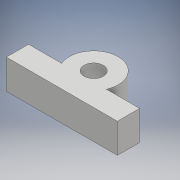
# Autodesk Inventor part: Mount for exis
Saved by Autodesk Inventor 2018 (Build 220112000, 112)
## iProperties
Created: 2019-04-02
Part Number: Mount for exis
Material: Типовые
Document SubType Name: Modeling
Designer: cosko
Density: 1 g/cm^3
Appearance: По умолчанию
Author: cosko
Autodesk Inventor part; units mm, degrees
ref_plane "YZ Plane" through (0, 0, 0) normal (1, 0, 0) x (0, 1, 0)
ref_plane "XZ Plane" through (0, 0, 0) normal (0, 1, 0) x (-1, 0, 0)
ref_plane "XY Plane" through (0, 0, 0) normal (0, 0, 1) x (1, 0, 0)
sketch "Эскиз1" plane through (0, 0, 0) normal (0, 0, 1) x (1, 0, 0)
  line L0 (0, 0) -> (0, 3) construction
  line L1 (0, 3) -> (2.6556, 3) construction
  line L2 (0, 3) -> (0, 5.6) construction
  circle A0 centre (0, 4.3) radius 1.3
  circle A1 centre (0, 4.3) radius 3.3
  line L3 (-7.5, 0) -> (7.5, 0)
  line L4 (7.5, 0) -> (7.5, 3)
  line L5 (7.5, 3) -> (-7.5, 3)
  line L6 (-7.5, 3) -> (-7.5, 0)
  line L7 (-7.5, 0) -> (7.5, 3) construction
  line L8 (7.5, 0) -> (-7.5, 3) construction
  point P0 (0, 1.5)
  dimension "d0" = 3
  dimension "d1" = 2.6
  dimension "d2" = 2
  dimension "d3" = 15
  dimension "d4" = 3
  constraints: 18 end point, 4 midpoint, 2 horizontal, 2 parallel, 2 vertical, 1 centre point, 1 perpendicular, 1 vertical alignment, 2 other
  measures "d0" distance of L0.start L0.end
  measures "d1" distance of L0.end L2.end
  measures "d3" distance of L5.end L4.end
  measures "d4" distance of L4.end L3.end
extrude "Выдавливание1" add sketch "Эскиз1" along normal blind 4
sketch "Эскиз3" plane through (-7.5, 3, 0) normal (0, 1, 0) x (1, 0, 0)
  line L0 (4.4668, 0) -> (4.4668, -4) projected
  line L1 (4.4668, 0) -> (0, 0) projected
  line L2 (0, 0) -> (0, -4) projected
  line L3 (4.4668, -4) -> (0, -4) projected
  circle A0 centre (2.2334, -2) radius 1.5
  line L4 (10.5332, -4) -> (10.5332, 0) projected
  line L5 (15, -4) -> (10.5332, -4) projected
  line L6 (15, 0) -> (15, -4) projected
  line L7 (15, 0) -> (10.5332, 0) projected
  circle A1 centre (12.7666, -2) radius 1.5
  point P0 (7.5, 0)
  dimension "d10" = 3
  dimension "d11" = 3
  constraints: 2 centre point
  measures "d10" diameter of A0
  measures "d11" diameter of A1
extrude "Выдавливание3" cut sketch "Эскиз3" against normal blind 2 contours A0 | A1
